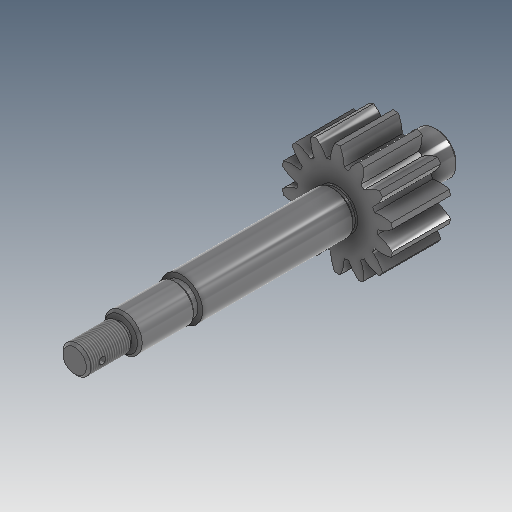
# Autodesk Inventor part: 主动齿轮轴
Saved by Autodesk Inventor 2020 (Build 240168000, 168)
## iProperties
Created: 2021-04-21
Part Number: 主动齿轮轴
Material: 钢
Document SubType Name: Modeling
Designer: Luorily
Density: 7.85 g/cm^3
Appearance: 氮化硅 - 抛光
Author: Luorily
Autodesk Inventor part; units mm, degrees
ref_plane "XY Plane" through (0, 0, 0) normal (0, 0, 1) x (1, 0, 0)
sketch "草图1" plane through (0, 0, 0) normal (0, 0, 1) x (1, 0, 0)
  circle A0 centre (0, 0) radius 9
  dimension "d0" = 18
  constraints: 1 centre point, 1 coincident
  measures "d0" diameter of A0
extrude "拉伸1" add sketch "草图1" along normal blind 16
sketch "草图2" plane through (0, 0, 16) normal (0, 0, 1) x (1, 0, 0)
  circle A0 centre (0, 0) radius 9 projected
  circle A1 centre (0, 0) radius 8.2
  dimension "d3" = 16.4
  constraints: 1 centre point, 1 coincident
  measures "d3" diameter of A1
extrude "拉伸2" add sketch "草图2" along normal blind 2 contours A1
sketch "草图3" plane through (0, 0, 18) normal (0, 0, 1) x (1, 0, 0)
  circle A0 centre (0, 0) radius 8.2 projected
  circle A1 centre (0, 0) radius 17.25
  dimension "d6" = 34.5
  constraints: 1 centre point, 1 coincident
  measures "d6" diameter of A1
extrude "拉伸3" add sketch "草图3" along normal blind 25 contours A0 | A1
sketch "草图4" plane through (0, 0, 43) normal (0, 0, 1) x (1, 0, 0)
  circle A0 centre (0, 0) radius 8.2 projected
  circle A1 centre (0, 0) radius 8.2
  constraints: 1 centre point, 1 coincident
extrude "拉伸4" add sketch "草图4" along normal blind 2
sketch "草图5" plane through (0, 0, 45) normal (0, 0, 1) x (1, 0, 0)
  circle A0 centre (0, 0) radius 8.2 projected
  circle A1 centre (0, 0) radius 9
  dimension "d11" = 18
  constraints: 1 centre point, 1 coincident
  measures "d11" diameter of A1
extrude "拉伸5" add sketch "草图5" along normal blind 65 contours A0 | A1
sketch "草图6" plane through (0, 0, 110) normal (0, 0, 1) x (1, 0, 0)
  circle A0 centre (0, 0) radius 9 projected
  circle A1 centre (0, 0) radius 7
  dimension "d14" = 14
  constraints: 1 centre point, 1 coincident
  measures "d14" diameter of A1
extrude "拉伸6" add sketch "草图6" along normal blind 2 contours A1
sketch "草图7" plane through (0, 0, 112) normal (0, 0, 1) x (1, 0, 0)
  circle A0 centre (0, 0) radius 7 projected
  circle A1 centre (0, 0) radius 8
  dimension "d17" = 16
  constraints: 1 centre point, 1 coincident
  measures "d17" diameter of A1
extrude "拉伸7" add sketch "草图7" along normal blind 24 contours A0 | A1
sketch "草图8" plane through (0, 0, 136) normal (0, 0, 1) x (1, 0, 0)
  circle A0 centre (0, 0) radius 7 projected
  circle A1 centre (0, 0) radius 4.5
  dimension "d20" = 9
  constraints: 1 centre point, 1 coincident
  measures "d20" diameter of A1
extrude "拉伸8" add sketch "草图8" along normal blind 2 contours A1
sketch "草图9" plane through (0, 0, 138) normal (0, 0, 1) x (1, 0, 0)
  circle A0 centre (0, 0) radius 7 projected
  circle A1 centre (0, 0) radius 6
  dimension "d23" = 12
  constraints: 1 centre point, 1 coincident
  measures "d23" diameter of A1
extrude "拉伸9" add sketch "草图9" along normal blind 18 contours A1
thread "螺纹2" size "M12x1" class "6g" standard "ANSI Metric M Profile" length 22
chamfer "倒角1" distance 1 angle 45 1 edges at (-6, 0, 156)
fillet "圆角2" radius 0.5 2 edges at (-8.2, 0, 16) (-8.2, 0, 18)
chamfer "倒角2" distance 0.3 angle 45 1 edges at (-9, 0, 16)
chamfer "倒角3" distance 0.3 angle 45 1 edges at (-9, 0, 45)
fillet "圆角4" radius 0.5 2 edges at (-8.2, 0, 45) (-8.2, 0, 43)
chamfer "倒角4" distance 1 angle 45 2 edges at (-8, 0, 112) (-8, 0, 136)
chamfer "倒角5" distance 1 angle 45 1 edges at (-9, 0, 0)
ref_plane "工作平面1" through (0, -3, 0) normal (0, 1, 0) x (-1, 0, 0)
sketch "草图11" plane through (0, -3, 0) normal (0, 1, 0) x (-1, 0, 0)
  line L0 (-7, 136) -> (7, 136) projected
  line L1 (0, 136) -> (0, 133)
  line L2 (0, 133) -> (0, 130.5)
  line L3 (0, 130.5) -> (0, 115.5)
  line L4 (0, 115.5) -> (0, 130.5) construction
  line L5 (-8, 113) -> (8, 113) projected
  line L6 (2.5, 115.5) -> (2.5, 130.5)
  line L7 (-2.5, 130.5) -> (-2.5, 115.5)
  arc A0 (-2.5, 115.5) -> (2.5, 115.5) centre (0, 115.5) ccw
  arc A1 (2.5, 130.5) -> (-2.5, 130.5) centre (0, 130.5) ccw
  point P0 (0, 0)
  point P1 (0, 123)
  dimension "d54" = 3
  dimension "d55" = 2.5
  dimension "d56" = 15
  dimension "d57" = 5
  constraints: 14 end point, 4 point on circle, 4 tangent, 2 centre point, 2 midpoint, 2 point on line, 1 parallel, 1 perpendicular, 1 vertical
  measures "d54" distance of L1.start L1.end
  measures "d55" distance of L1.end L2.end
  measures "d56" distance of L2.end L3.end
  measures "d57" diameter of A1
extrude "拉伸10" cut sketch "草图11" against normal blind 18
ref_plane "工作平面2" through (-6, 0, 138) normal (1, 0, 0) x (0, 1, 0)
sketch "草图12" plane through (-6, 0, 138) normal (1, 0, 0) x (0, 1, 0)
  line L0 (-5, 18) -> (5, 18) projected
  line L1 (0, 18) -> (0, 12)
  point P0 (0, -138)
  dimension "d60" = 6
  constraints: 2 end point, 1 coincident, 1 midpoint, 1 vertical
  measures "d60" distance of L1.start L1.end
hole "孔1" at (-6, 0, 150) direction (1, 0, 0) diameter 2.85 end through all thread size "M3.5x0.6" designation "M3.5" class "6H" standard "GB Metric profile"
sketch "草图13" plane through (0, 0, 18) normal (0, 0, -1) x (-1, 0, 0)
  circle A0 centre (0, 0) radius 17.25 projected
  circle A1 centre (0, 0) radius 8.7 projected
  circle A2 centre (0, 0) radius 21
  circle A3 centre (0, 0) radius 24
  circle A4 centre (0, 0) radius 17.25 projected
  arc A5 (-1.1074, 23.9744) -> (-2.8831, 17.0074) centre (11.9993, 16.9242) ccw
  line L0 (0, 0) -> (0, 27.2026) construction
  arc A6 (2.8831, 17.0074) -> (1.1074, 23.9744) centre (-11.9993, 16.9242) ccw
  arc A7 (1.1074, 23.9744) -> (-1.1074, 23.9744) centre (0, 0) ccw
  point P0 (-2.3513, 20.868)
  point P1 (2.3513, 20.868)
  point P2 (2.8831, 17.0074)
  point P3 (-2.8831, 17.0074)
  dimension "d68" = 42
  dimension "d69" = 48
  dimension "d70" = 12.857
  constraints: 13 point on circle, 5 centre point, 3 symmetric about line, 2 coincident, 2 end point, 1 vertical, 3 other
  measures "d68" diameter of A2
  measures "d69" diameter of A3
extrude "拉伸11" add sketch "草图13" against normal up to surface (25 mm away) contours A0 A5 A2 A6 | A2 A5 A3 A6 picked at (-0.2617, 18.4771) picked at (0.1231, 21.9893)
pattern_circular "环形阵列1" count 14 over 360 about axis through (0, 0, 18) along (0, 0, 1) of "拉伸11"
